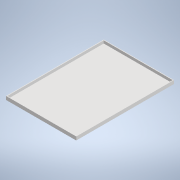
# Autodesk Inventor part: trayCover
Saved by Autodesk Inventor 2022 (Build 260153000, 153)
## iProperties
Created: 2023-05-08
Part Number: trayCover
Material: Generic
Document SubType Name: Modeling
Designer: Hallgato
Density: 1 g/cm^3
Appearance: Default
Author: Hallgato
Autodesk Inventor part; units mm, degrees
ref_plane "YZ Plane" through (0, 0, 0) normal (1, 0, 0) x (0, 1, 0)
ref_plane "XZ Plane" through (0, 0, 0) normal (0, 1, 0) x (-1, 0, 0)
ref_plane "XY Plane" through (0, 0, 0) normal (0, 0, 1) x (1, 0, 0)
sketch "Sketch1" plane through (0, 0, 0) normal (0, 1, 0) x (-1, 0, 0)
  circle A0 centre (0, 0) radius 19.4
  line L0 (0, 0) -> (0, -10.9961) construction
  circle A1 centre (0, -45) radius 19.4
  circle A2 centre (45, 22.5) radius 19.4
  circle A3 centre (45, -22.5) radius 19.4
  circle A4 centre (45, -67.5) radius 19.4
  line L1 (-27.5, -92.5) -> (72.5, -92.5)
  line L2 (72.5, -92.5) -> (72.5, 47.5)
  line L3 (72.5, 47.5) -> (-27.5, 47.5)
  line L4 (-27.5, 47.5) -> (-27.5, -92.5)
  line L5 (-27.5, -92.5) -> (72.5, 47.5) construction
  line L6 (72.5, -92.5) -> (-27.5, 47.5) construction
  line L7 (73.5, 48.5) -> (-28.5, 48.5)
  line L8 (-28.5, 48.5) -> (-28.5, -93.5)
  line L9 (-28.5, -93.5) -> (73.5, -93.5)
  line L10 (73.5, -93.5) -> (73.5, 48.5)
  point P0 (22.5, -22.5)
  dimension "d0" = 38.8
  dimension "d3" = 45
  dimension "d8" = 38.8
  dimension "d9" = 45
  dimension "d10" = 22.5
  dimension "d13" = 45
  dimension "d18" = 22.5
  dimension "d19" = 50
  dimension "d20" = 70
  dimension "d21" = 22.5
  dimension "d37" = 1
  dimension "d38" = 1
  dimension "d39" = 1
  dimension "d40" = 1
  constraints: 22 end point, 5 centre point, 4 parallel, 3 vertical, 2 horizontal, 2 midpoint, 2 perpendicular, 1 coincident, 6 other
  measures "d0" diameter of A0
  measures "d3" distance of L0.start A1.centre
  measures "d8" diameter of A2
  measures "d9" horizontal distance of A2.centre point (0, 0)
  measures "d10" vertical distance of point (0, 0) A2.centre
  measures "d13" distance of A2.centre A3.centre
  measures "d18" distance of point (22.5, -22.5) A3.centre
  measures "d19" distance from line of L4 point (22.5, -22.5)
  measures "d20" distance from line of L1 point (22.5, -22.5)
  measures "d21" horizontal distance of point (22.5, -22.5) A1.centre
  measures "d37" distance between parallel lines of L7 L3
  measures "d38" distance between parallel lines of L8 L4
  measures "d39" distance between parallel lines of L9 L1
  measures "d40" distance between parallel lines of L2 L10
extrude "Extrusion4" add sketch "Sketch1" against normal blind 1 contours A0 | A1 | A2 | A3 | A4 | L4 L3 L2 L1 | L10 L9 L8 L7
extrude "Extrusion5" add sketch "Sketch1" along normal blind 4 contours L10 L9 L8 L7
equation "\"d0\" = bottleDiameter"
equation "\"d3\" = bottleDistance"
equation "\"d8\" = bottleDiameter"
equation "\"d9\" = bottleDistance"
equation "\"d10\" = 0.5 * bottleDistance"
equation "\"d13\" = bottleDistance"
equation "\"d18\" = 0.5 * bottleDistance"
equation "\"d21\" = 0.5 * bottleDistance"
equation "\"d37\" = tpuTick"
equation "\"d38\" = tpuTick"
equation "\"d39\" = tpuTick"
equation "\"d40\" = tpuTick"
equation "\"d41\" = tpuTick"
equation "\"capDiameter\" = 29.5"
equation "\"bottleLen\" = 81.3"
equation "\"bottleDiameter\" = 38.8"
equation "\"tubeInsideDiameter\" = 2"
equation "\"tubeOutsideDiameter\" = 5.4"
equation "\"tick\" = 2"
equation "\"connectorDiameter\" = 35"
equation "\"connectorInsideDiameter\" = tubeInsideDiameter - tick"
equation "\"connectorTubeDepth\" = 18.5"
equation "\"tubeFlapDepth\" = 3"
equation "\"tubeFlapAngle\" = 15deg"
equation "\"minTick\" = 0.25"
equation "\"tubeLinkTick\" = 2"
equation "\"tubeTolerance\" = 0.3"
equation "\"tickHolder\" = 1"
equation "\"bottleDistance\" = 45"
equation "\"tpuTick\" = 1"
body "Solid2"
